18 teath (Autodesk Fusion 360 design; units mm, degrees)
description: Spur Gear; Module: 1.27; Num Teeth: 18; Pressure Angle: 20.0; Backlash: 0.00 mm
part number: 2026-06-12-03-24-41-534
Autodesk Fusion 360 part; units mm, degrees
sketch "Base Circle" plane through (0, 0, 0) normal (0, 0, 1) x (1, 0, 0)
  circle A0 centre (0, 0) radius 9.9606
  circle A1 centre (0, 0) radius 2.5
extrude "Extrude1" add sketch "Base Circle" along normal blind 1
sketch "Gear Tooth" plane through (0, 0, 0) normal (0, 0, 1) x (1, 0, 0)
  spline S0 degree 5 poles (10.6847, -1.0955) (10.6904, -1.0961) (10.7018, -1.0971) (10.719, -1.0981) (10.7419, -1.0986) (10.7706, -1.098) (10.7994, -1.0966) (10.8282, -1.0945) (10.8571, -1.0922) (10.8859, -1.0897) (10.9148, -1.0869) (10.9437, -1.0839) (10.9726, -1.0805) (11.0015, -1.0767) (11.0304, -1.0724) (11.0594, -1.0678) (11.0883, -1.0628) (11.1173, -1.0575) (11.1462, -1.052) (11.1752, -1.0462) (11.2042, -1.0402) (11.2331, -1.0339) (11.2621, -1.0274) (11.2911, -1.0205) (11.32, -1.0135) (11.349, -1.0061) (11.3779, -0.9986) (11.4069, -0.9907) (11.4358, -0.9827) (11.4647, -0.9744) (11.4937, -0.9659) (11.5226, -0.9572) (11.5515, -0.9483) (11.5804, -0.9391) (11.6093, -0.9298) (11.6381, -0.9202) (11.667, -0.9104) (11.6959, -0.9004) (11.7247, -0.8902) (11.7535, -0.8798) (11.7823, -0.8691) (11.8111, -0.8583) (11.8399, -0.8473) (11.8686, -0.8361) (11.8974, -0.8247) (11.9261, -0.8132) (11.9548, -0.8014) (11.9835, -0.7894) (12.0121, -0.7773) (12.0408, -0.7649) (12.0694, -0.7524) (12.098, -0.7397) (12.1266, -0.7268) (12.1551, -0.7138) (12.1837, -0.7005) (12.2122, -0.6871) (12.2407, -0.6735) (12.2691, -0.6597) (12.2976, -0.6458) (12.326, -0.6317) (12.3543, -0.6174) (12.3827, -0.6029) (12.411, -0.5883) (12.4393, -0.5735) (12.4676, -0.5585) (12.4958, -0.5434) (12.524, -0.5281) (12.5522, -0.5126) (12.5804, -0.497) (12.6085, -0.4812) (12.6366, -0.4652) (12.659, -0.4523) (12.6758, -0.4426) (12.687, -0.436) (12.6926, -0.4328) knots 0 0 0 0 0 0 0.01428571 0.02857143 0.04285714 0.05714286 0.07142857 0.08571429 0.1 0.11428571 0.12857143 0.14285714 0.15714286 0.17142857 0.18571429 0.2 0.21428571 0.22857143 0.24285714 0.25714286 0.27142857 0.28571429 0.3 0.31428571 0.32857143 0.34285714 0.35714286 0.37142857 0.38571429 0.4 0.41428571 0.42857143 0.44285714 0.45714286 0.47142857 0.48571429 0.5 0.51428571 0.52857143 0.54285714 0.55714286 0.57142857 0.58571429 0.6 0.61428571 0.62857143 0.64285714 0.65714286 0.67142857 0.68571429 0.7 0.71428571 0.72857143 0.74285714 0.75714286 0.77142857 0.78571429 0.8 0.81428571 0.82857143 0.84285714 0.85714286 0.87142857 0.88571429 0.9 0.91428571 0.92857143 0.94285714 0.95714286 0.97142857 0.98571429 1 1 1 1 1 1
  spline S1 degree 5 poles (10.6847, 1.0955) (10.6904, 1.0961) (10.7018, 1.0971) (10.719, 1.0981) (10.7419, 1.0986) (10.7706, 1.098) (10.7994, 1.0966) (10.8282, 1.0945) (10.8571, 1.0922) (10.8859, 1.0897) (10.9148, 1.0869) (10.9437, 1.0839) (10.9726, 1.0805) (11.0015, 1.0767) (11.0304, 1.0724) (11.0594, 1.0678) (11.0883, 1.0628) (11.1173, 1.0575) (11.1462, 1.052) (11.1752, 1.0462) (11.2042, 1.0402) (11.2331, 1.0339) (11.2621, 1.0274) (11.2911, 1.0205) (11.32, 1.0135) (11.349, 1.0061) (11.3779, 0.9986) (11.4069, 0.9907) (11.4358, 0.9827) (11.4647, 0.9744) (11.4937, 0.9659) (11.5226, 0.9572) (11.5515, 0.9483) (11.5804, 0.9391) (11.6093, 0.9298) (11.6381, 0.9202) (11.667, 0.9104) (11.6959, 0.9004) (11.7247, 0.8902) (11.7535, 0.8798) (11.7823, 0.8691) (11.8111, 0.8583) (11.8399, 0.8473) (11.8686, 0.8361) (11.8974, 0.8247) (11.9261, 0.8132) (11.9548, 0.8014) (11.9835, 0.7894) (12.0121, 0.7773) (12.0408, 0.7649) (12.0694, 0.7524) (12.098, 0.7397) (12.1266, 0.7268) (12.1551, 0.7138) (12.1837, 0.7005) (12.2122, 0.6871) (12.2407, 0.6735) (12.2691, 0.6597) (12.2976, 0.6458) (12.326, 0.6317) (12.3543, 0.6174) (12.3827, 0.6029) (12.411, 0.5883) (12.4393, 0.5735) (12.4676, 0.5585) (12.4958, 0.5434) (12.524, 0.5281) (12.5522, 0.5126) (12.5804, 0.497) (12.6085, 0.4812) (12.6366, 0.4652) (12.659, 0.4523) (12.6758, 0.4426) (12.687, 0.436) (12.6926, 0.4328) knots 0 0 0 0 0 0 0.01428571 0.02857143 0.04285714 0.05714286 0.07142857 0.08571429 0.1 0.11428571 0.12857143 0.14285714 0.15714286 0.17142857 0.18571429 0.2 0.21428571 0.22857143 0.24285714 0.25714286 0.27142857 0.28571429 0.3 0.31428571 0.32857143 0.34285714 0.35714286 0.37142857 0.38571429 0.4 0.41428571 0.42857143 0.44285714 0.45714286 0.47142857 0.48571429 0.5 0.51428571 0.52857143 0.54285714 0.55714286 0.57142857 0.58571429 0.6 0.61428571 0.62857143 0.64285714 0.65714286 0.67142857 0.68571429 0.7 0.71428571 0.72857143 0.74285714 0.75714286 0.77142857 0.78571429 0.8 0.81428571 0.82857143 0.84285714 0.85714286 0.87142857 0.88571429 0.9 0.91428571 0.92857143 0.94285714 0.95714286 0.97142857 0.98571429 1 1 1 1 1 1
  arc A0 (12.6926, -0.4328) -> (12.6926, 0.4328) centre (0, 0) ccw
  line L0 (9.8987, -1.0149) -> (10.6847, -1.0955)
  line L1 (9.8987, 1.0149) -> (10.6847, 1.0955)
  line L2 (9.8987, -1.0149) -> (9.8987, 1.0149)
  point P0 (10.8254, -1.0947)
  point P1 (10.9674, -1.081)
  point P2 (11.1102, -1.0588)
  point P3 (11.2535, -1.0293)
  point P4 (11.3972, -0.9933)
  point P5 (11.5412, -0.9514)
  point P6 (11.6854, -0.904)
  point P7 (11.8297, -0.8512)
  point P8 (11.974, -0.7934)
  point P9 (12.1182, -0.7306)
  point P10 (12.2622, -0.663)
  point P11 (12.406, -0.5908)
  point P12 (12.5495, -0.514)
  point P13 (10.8254, 1.0947)
  point P14 (10.9674, 1.081)
  point P15 (11.1102, 1.0588)
  point P16 (11.2535, 1.0293)
  point P17 (11.3972, 0.9933)
  point P18 (11.5412, 0.9514)
  point P19 (11.6854, 0.904)
  point P20 (11.8297, 0.8512)
  point P21 (11.974, 0.7934)
  point P22 (12.1182, 0.7306)
  point P23 (12.2622, 0.663)
  point P24 (12.406, 0.5908)
  point P25 (12.5495, 0.514)
extrude "Extrude2" add sketch "Gear Tooth" along normal blind 1
fillet "Fillet1" radius 0.2 2 edges at (9.9087, -1.0159, 0.5) (9.9087, 1.0159, 0.5)
pattern_circular "C-Pattern1" count 18 over 360 about axis through (0, 0, 0) along (0, 0, 1) of "Extrude2", "Fillet1"
sketch "Diametrial Pitch Circle" plane through (0, 0, 0) normal (0, 0, 1) x (1, 0, 0)
  circle A0 centre (0, 0) radius 11.43 construction
extrude "Extrude3" add 1 faces at (7.4358, 0, 0) along direction (0, 0, -1) blind 2
named bodies: "Spur Gear (18 teeth)"
